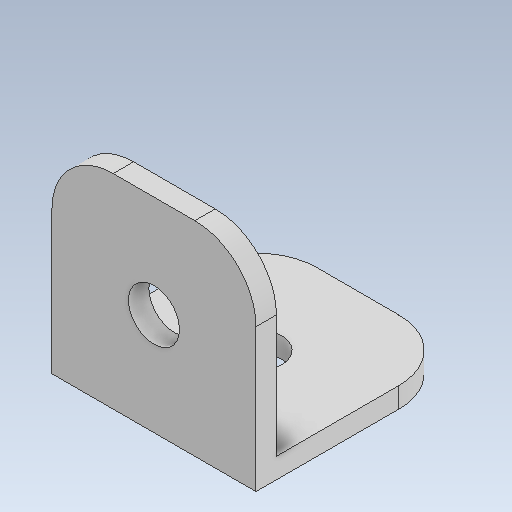
# Autodesk Inventor part: 80-20 bracket 1in
Saved by Autodesk Inventor 2020.2 (Build 242310000, 310)
## iProperties
Created: 2020-02-02
Part Number: 80-20 bracket 1in
Material: Generic
Document SubType Name: Modeling
Designer: lucas
Density: 1 g/cm^3
Appearance: Default
Mass: 2.82606 g
Surface Area: 26.6755 cm^2
Volume: 2.82606 cm^3
Author: lucas
Autodesk Inventor part; units mm, degrees
ref_plane "YZ Plane" through (0, 0, 0) normal (1, 0, 0) x (0, 1, 0)
ref_plane "XZ Plane" through (0, 0, 0) normal (0, 1, 0) x (-1, 0, 0)
ref_plane "XY Plane" through (0, 0, 0) normal (0, 0, 1) x (1, 0, 0)
sketch "Sketch1" plane through (0, 0, 0) normal (1, 0, 0) x (0, 1, 0)
  line L0 (-21.9539, 18.6933) -> (3.4461, 18.6933)
  line L1 (3.4461, 18.6933) -> (3.4461, 21.2333)
  line L2 (3.4461, 21.2333) -> (-21.9539, 21.2333)
  line L3 (-21.9539, 21.2333) -> (-21.9539, 18.6933)
  line L4 (-21.9539, 18.6933) -> (-19.4139, 18.6933)
  line L5 (-19.4139, 18.6933) -> (-19.4139, -4.1667)
  line L6 (-19.4139, -4.1667) -> (-21.9539, -4.1667)
  line L7 (-21.9539, -4.1667) -> (-21.9539, 18.6933)
  point P0 (0, 0)
  dimension "d0" = 2.54
  dimension "d1" = 2.54
  dimension "d2" = 25.4
  dimension "d3" = 25.4
  constraints: 16 end point, 4 parallel, 2 horizontal, 2 perpendicular
  measures "d0" distance of L5.end L6.end
  measures "d1" distance of L0.end L1.end
  measures "d2" distance of L1.end L2.end
  measures "d3" distance between parallel lines of L2 L6
extrude "Extrusion1" add sketch "Sketch1" along normal blind 25.4
sketch "Sketch2" plane through (0, -21.9539, 21.2333) normal (0, 0, 1) x (1, 0, 0)
  circle A0 centre (12.7, 12.7) radius 3.175
  line L0 (0, 25.4) -> (25.4, 25.4) projected
  line L1 (25.4, 25.4) -> (25.4, 0) projected
  point P0 (0, 21.9539)
  dimension "d6" = 6.35
  dimension "d7" = 12.7
  dimension "d8" = 12.7
  constraints: 1 centre point
  measures "d6" diameter of A0
  measures "d7" distance from line of L0 A0.centre
  measures "d8" distance from line of L1 A0.centre
extrude "Extrusion2" cut sketch "Sketch2" against normal blind 25.4
sketch "Sketch3" plane through (0, -21.9539, -4.1667) normal (0, -1, 0) x (1, 0, 0)
  circle A0 centre (12.7, 12.7) radius 3.175
  line L0 (0, 25.4) -> (25.4, 25.4) projected
  line L1 (25.4, 25.4) -> (25.4, 0) projected
  point P0 (0, 4.1667)
  dimension "d11" = 12.7
  dimension "d12" = 12.7
  dimension "d13" = 6.35
  constraints: 1 centre point
  measures "d11" distance from line of L0 A0.centre
  measures "d12" distance from line of L1 A0.centre
  measures "d13" diameter of A0
extrude "Extrusion3" cut sketch "Sketch3" against normal blind 25.4
fillet "Fillet1" radius 7.62 4 edges at (25.4, 3.4461, 19.9633) (0, 3.4461, 19.9633) (25.4, -20.6839, -4.1667) (0, -20.6839, -4.1667)
body "Solid1"
